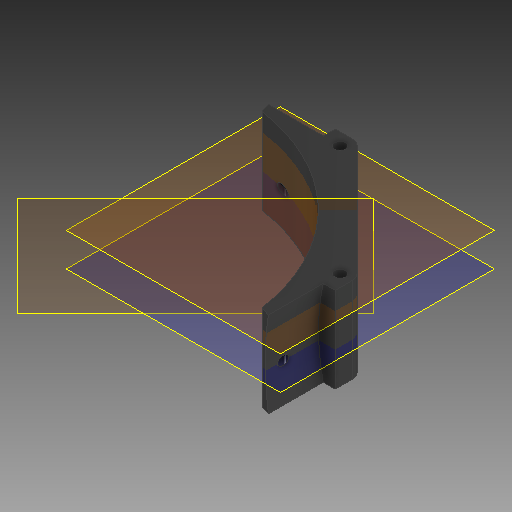
# Autodesk Inventor part: сфеср
Saved by Autodesk Inventor 2020 (Build 240168000, 168)
## iProperties
Created: 2024-09-14
Part Number: сфеср
Material: Типовые
Document SubType Name: Modeling
Designer: Ivan
Density: 1 g/cm^3
Appearance: Черный — литой
Author: Ivan
Autodesk Inventor part; units mm, degrees
ref_plane "YZ Plane" through (0, 0, 0) normal (1, 0, 0) x (0, 1, 0)
ref_plane "XZ Plane" through (0, 0, 0) normal (0, 1, 0) x (-1, 0, 0)
ref_plane "XY Plane" through (0, 0, 0) normal (0, 0, 1) x (1, 0, 0)
sketch "Эскиз1" plane through (0, 0, 0) normal (0, 1, 0) x (-1, 0, 0)
  circle A0 centre (-44.87, 82.9015) radius 1.5
  line L0 (-31, 99.2724) -> (-31, 78.7724)
  line L1 (-31, 78.7724) -> (31, 78.7724)
  circle A1 centre (-42.22, 16) radius 1.5
  circle A2 centre (-16, 42.22) radius 1.5
  circle A3 centre (16, 42.22) radius 1.5
  circle A4 centre (31, 72.43) radius 1.5
  circle A5 centre (16, 72.43) radius 1.5
  circle A6 centre (-16, 72.43) radius 1.5
  arc A7 (-31, 99.2724) -> (-99.2724, 31) centre (0, 0) ccw
  circle A8 centre (-74.5664, 57.67) radius 1.5
  circle A9 centre (-82.9015, 44.87) radius 1.5
  circle A10 centre (-72.43, -16) radius 1.5
  circle A11 centre (-72.43, 16) radius 1.5
  line L2 (-78.7724, 31) -> (-78.7724, -31)
  line L3 (-99.2724, 31) -> (-78.7724, 31)
  line L4 (31, 78.7724) -> (31, 99.2724)
  arc A12 (34.57, 98.0863) -> (98.0863, 34.57) centre (109.0212, 109.0212) ccw
  circle A13 centre (72.43, 31) radius 1.5
  line L5 (99.2724, 31) -> (78.7724, 31)
  circle A14 centre (72.43, 16) radius 1.5
  arc A15 (34.57, 98.0863) -> (31, 99.2724) centre (0, 0) ccw
  arc A16 (99.2724, 31) -> (98.0863, 34.57) centre (0, 0) ccw
  arc A17 (98.0863, 34.57) -> (34.57, 98.0863) centre (0, 0) ccw
  circle A18 centre (42.22, 16) radius 1.5
  circle A19 centre (82.9015, -44.87) radius 1.5
  line L6 (78.7724, -31) -> (99.2724, -31)
  arc A20 (31, -99.2724) -> (99.2724, -31) centre (0, 0) ccw
  circle A21 centre (16, -72.43) radius 1.5
  line L7 (31, -78.7724) -> (31, -99.2724)
  circle A22 centre (44.87, -82.9015) radius 1.5
  circle A23 centre (57.67, -74.5664) radius 1.5
  circle A24 centre (-57.67, 74.5664) radius 1.5
  circle A25 centre (-42.22, -16) radius 1.5
  circle A26 centre (42.22, -16) radius 1.5
  circle A27 centre (-72.43, -31) radius 1.5
  line L8 (-73.5391, 73.5391) -> (73.5391, -73.5391) construction
  line L9 (78.7724, 31) -> (78.7724, -31)
  circle A28 centre (72.43, -16) radius 1.5
  circle A29 centre (-16, -42.22) radius 1.5
  circle A30 centre (16, -42.22) radius 1.5
  circle A31 centre (74.5664, -57.67) radius 1.5
  line L10 (-31, -78.7724) -> (31, -78.7724)
  circle A32 centre (-16, -72.43) radius 1.5
  circle A33 centre (-31, -72.43) radius 1.5
  line L11 (-31, -99.2724) -> (-31, -78.7724)
  arc A34 (-34.57, -98.0863) -> (-31, -99.2724) centre (0, 0) ccw
  line L12 (-78.7724, -31) -> (-99.2724, -31)
  arc A35 (-99.2724, -31) -> (-98.0863, -34.57) centre (0, 0) ccw
  arc A36 (-98.0863, -34.57) -> (-34.57, -98.0863) centre (0, 0) ccw
  arc A37 (-34.57, -98.0863) -> (-98.0863, -34.57) centre (-109.0212, -109.0212) ccw
  constraints: 38 centre point, 26 end point, 23 point on circle, 5 coincident, 1 horizontal, 1 perpendicular, 1 symmetric about line, 2 other
sketch "Эскиз2" plane through (0, 0, 0) normal (0, 1, 0) x (-1, 0, 0)
  arc A0 (34.57, 98.0863) -> (98.0863, 34.57) centre (109.0212, 109.0212) ccw projected
  arc A1 (99.2724, 31) -> (98.0863, 34.57) centre (0, 0) ccw projected
  arc A2 (34.57, 98.0863) -> (31, 99.2724) centre (0, 0) ccw projected
  line L0 (31, 78.7724) -> (31, 99.2724) projected
  circle A3 centre (31, 72.43) radius 1.5 projected
  circle A4 centre (72.43, 31) radius 1.5 projected
  circle A5 centre (31, 72.43) radius 4.5
  circle A6 centre (72.43, 31) radius 4.5
  line L1 (27.818, 69.248) -> (69.248, 27.818)
  line L2 (26.5, 78.7724) -> (26.5, 72.43)
  line L3 (78.7724, 31) -> (78.7724, -31) projected
  line L4 (78.7724, 26.5) -> (72.43, 26.5)
  line L5 (99.2724, 31) -> (78.7724, 31) projected
  line L6 (26.5, 78.7724) -> (31, 78.7724)
  dimension "d0" = 9
  dimension "d1" = 9
  constraints: 8 end point, 4 point on circle, 4 tangent, 2 centre point, 2 coincident, 2 horizontal, 1 point on line, 1 vertical
  measures "d0" diameter of A5
  measures "d1" diameter of A6
extrude "Выдавливание1" add sketch "Эскиз2" along normal blind 32
ref_plane "РабПлоскость1" through (0, 25.3, 0) normal (0, 1, 0) x (1, 0, 0)
sketch "Эскиз3" plane through (0, 25.3, 0) normal (0, 1, 0) x (1, 0, 0)
  circle A0 centre (-72.43, -31) radius 1.5 projected
  circle A1 centre (-31, -72.43) radius 1.5 projected
  point P0 (0, 0)
extrude "Выдавливание2" add sketch "Эскиз3" against normal blind 20.6
sketch "Эскиз4" plane through (-31, 0, 78.7724) normal (0, 0, 1) x (1, 0, 0)
  line L0 (0, 1) -> (0, 32)
  line L1 (0, 32) -> (-3.57, 32) projected
  line L2 (0, 0) -> (0, 32) projected
  arc A0 (0, 32) -> (0, 0) centre (72.5929, 16) ccw
  point P0 (31, 0)
  constraints: 2 end point, 2 point on circle, 1 centre point, 1 vertical
extrude "Выдавливание3" cut sketch "Эскиз4" along normal through all
ref_plane "РабПлоскость2" through (-48.533, 0, 48.533) normal (0.7071068, 0, 0.7071068) x (0, 1, 0)
mirror "Зеркальное отражение1" about plane through (-48.533, 0, 48.533) normal (0.7071068, 0, 0.7071068) of "Выдавливание3"
sketch "Эскиз6" plane through (0, 0, 0) normal (0, 1, 0) x (1, 0, 0)
  circle A0 centre (124.1994, 64.0459) radius 3
  circle A1 centre (-31, -72.43) radius 1.5 projected
  circle A2 centre (-72.43, -31) radius 1.5 projected
  line L0 (-72.43, -31) -> (-31, -72.43)
  line L1 (-31, -72.43) -> (-36.2927, -77.7227)
  circle A3 centre (-36.2927, -77.7227) radius 2
  line L2 (164.6688, 164.6688) -> (-154.6363, -154.6363) projected
  circle A4 centre (-77.7227, -36.2927) radius 2
  point P0 (0, 0)
  point P1 (129.0863, 44.2024)
  dimension "d12" = 6
  dimension "d13" = 7.485
  dimension "d14" = 4
  constraints: 4 end point, 3 centre point, 1 coincident, 1 perpendicular, 1 symmetric about line, 1 other
  measures "d12" diameter of A0
  measures "d13" distance from line of L0 L1.end
  measures "d14" diameter of A3
extrude "Выдавливание5" cut sketch "Эскиз6" along normal blind 7 contours A3 | A4
ref_plane "РабПлоскость4" through (0, 12.8, 0) normal (0, -1, 0) x (1, 0, 0)
sketch "Эскиз9" plane through (0, 12.8, 0) normal (0, -1, 0) x (1, 0, 0)
  line L0 (-83.2724, 34) -> (-96.2724, 34)
  line L1 (-96.2724, 34) -> (-96.2724, 31)
  line L2 (-96.2724, 31) -> (-83.2724, 31)
  line L3 (-83.2724, 31) -> (-83.2724, 34)
  line L4 (-99.2724, 31) -> (-78.7724, 31)
  point P0 (0, 0)
  point P1 (0, 0)
  dimension "d23" = 3
  dimension "d24" = 13
  dimension "d43" = 3
  constraints: 10 end point, 3 parallel, 1 perpendicular, 1 point on line
  measures "d23" distance from line of L2 L0.start
  measures "d24" distance from line of L1 L2.end
  measures "d43" distance of L4.start L1.end
extrude "Выдавливание6" cut sketch "Эскиз9" along normal mid plane 5.15
sketch "Эскиз10" plane through (-48.533, 0, 48.533) normal (0.7071068, 0, 0.7071068) x (0, 1, 0)
  line L0 (15.375, 14.288) -> (10.225, 14.288) projected
  line L1 (12.8, 14.288) -> (12.8, 27.3139)
  circle A0 centre (12.8, 19.5665) radius 1.5
  line L2 (0, 5.8027) -> (32, 5.8027) projected
  point P0 (0, -68.6361)
  dimension "d29" = 3
  dimension "d31" = 13.7638
  constraints: 2 end point, 1 centre point, 1 midpoint, 1 point on line, 1 vertical
  measures "d29" diameter of A0
  measures "d31" distance from line of L2 A0.centre
extrude "Выдавливание7" cut sketch "Эскиз10" along normal mid plane 100
hole "Отверстие1" at (-72.43, 0, 31) at (-31, 0, 72.43) direction (0, 1, 0) diameter 4 depth 4.7
sketch "Эскиз11" plane through (0, 32, 0) normal (0, 1, 0) x (1, 0, 0)
  circle A0 centre (-72.43, -31) radius 1.5 projected
  circle A1 centre (-31, -72.43) radius 1.5 projected
  circle A2 centre (-72.43, -31) radius 2 projected
  circle A3 centre (-31, -72.43) radius 2 projected
  point P0 (0, 0)
  constraints: 2 coincident
extrude "Выдавливание8" cut sketch "Эскиз11" against normal up to surface (6.7 mm away) contours A0 | A1 | A2 | A3
equation "\"d1\" = d0"
